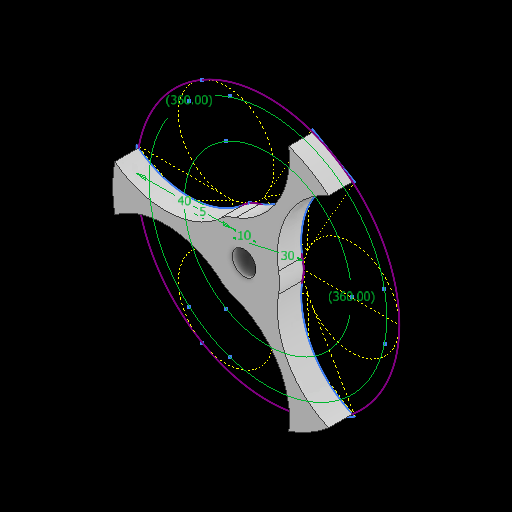
# Autodesk Inventor part: Combine mk1
Saved by Autodesk Inventor 2025 (Build 290162000, 162)
## iProperties
Created: 2024-09-10
Part Number: Combine mk1
Material: Generic
Document SubType Name: Modeling
Designer: Trevor
Density: 1 g/cm^3
Appearance: Default
Author: Trevor
Autodesk Inventor part; units mm, degrees
ref_plane "YZ Plane" through (0, 0, 0) normal (1, 0, 0) x (0, 1, 0)
ref_plane "XZ Plane" through (0, 0, 0) normal (0, 1, 0) x (-1, 0, 0)
ref_plane "XY Plane" through (0, 0, 0) normal (0, 0, 1) x (1, 0, 0)
sketch "Sketch1" plane through (0, 0, 0) normal (0, 0, 1) x (1, 0, 0)
  circle A0 centre (0, 0) radius 15
  circle A1 centre (0, 0) radius 55
  line L0 (15, 0) -> (55, 0) construction
  circle A2 centre (35, 0) radius 20 construction
  circle A3 centre (-17.5, 30.310889) radius 20 construction
  circle A4 centre (-17.5, -30.310889) radius 20 construction
  line L1 (0, 0) -> (-10.833994, 10.374226)
  line L2 (0, 0) -> (27.5, -47.631397)
  line L3 (0, 0) -> (-55, 0) construction
  line L4 (0, 0) -> (27.5, 47.631397)
  line L5 (17.5, 30.310889) -> (27.5, 47.631397) construction
  line L6 (-1.432373, 18.147489) -> (18.567627, 52.788505) construction
  line L7 (18.567627, 52.788505) -> (36.432373, 42.47429) construction
  line L8 (36.432373, 42.47429) -> (16.432373, 7.833273) construction
  line L9 (16.432373, 7.833273) -> (-1.432373, 18.147489) construction
  line L10 (-1.432373, 18.147489) -> (36.432373, 42.47429) construction
  line L11 (18.567627, 52.788505) -> (16.432373, 7.833273) construction
  line L12 (-1.48905, -18.180212) -> (18.51095, -52.821228) construction
  line L13 (18.51095, -52.821228) -> (36.48905, -42.441567) construction
  line L14 (36.48905, -42.441567) -> (16.48905, -7.80055) construction
  line L15 (16.48905, -7.80055) -> (-1.48905, -18.180212) construction
  line L16 (-1.48905, -18.180212) -> (36.48905, -42.441567) construction
  line L17 (18.51095, -52.821228) -> (16.48905, -7.80055) construction
  line L18 (-55.008072, 10.310889) -> (-15, 10.310889) construction
  line L19 (-15, 10.310889) -> (-15, -10.310889) construction
  line L20 (-15, -10.310889) -> (-55.008072, -10.310889) construction
  line L21 (-55.008072, -10.310889) -> (-55.008072, 10.310889)
  line L22 (-55.008072, 10.310889) -> (-15, -10.310889) construction
  line L23 (-15, 10.310889) -> (-55.008072, -10.310889) construction
  line L24 (-39.117828, -2.5) -> (-30.890244, -2.5) construction
  line L25 (-30.890244, -2.5) -> (-30.890244, 2.5) construction
  line L26 (-30.890244, 2.5) -> (-39.117828, 2.5) construction
  line L27 (-39.117828, 2.5) -> (-39.117828, -2.5) construction
  line L28 (-39.117828, -2.5) -> (-30.890244, 2.5) construction
  line L29 (-30.890244, -2.5) -> (-39.117828, 2.5) construction
  arc A5 (-10.89429, -10.310889) -> (-55.008072, -10.310889) centre (-32.951181, -37.548278) ccw
  line L30 (-55.008072, 10.310889) -> (-55.008072, -10.310889) construction
  arc A6 (-55.008072, 10.310889) -> (-10.833994, 10.374226) centre (-32.959623, 37.256893) ccw
  line L31 (-55.008072, 10.310889) -> (-55.008072, -10.310889) construction
  arc A7 (18.574544, -52.793832) -> (-3.567347, -14.569627) centre (-15.785604, -47.172317) ccw
  line L32 (36.433528, -42.482943) -> (18.574544, -52.793832)
  arc A8 (14.376637, -4.279288) -> (36.433528, -42.482943) centre (48.993353, -9.762421) ccw
  circle A9 centre (0, 0) radius 15
  arc A10 (36.433528, 42.482943) -> (14.401341, 4.195401) centre (48.745227, 9.915425) ccw
  line L33 (18.574544, 52.793832) -> (36.433528, 42.482943)
  arc A11 (-3.482347, 14.590177) -> (18.574544, 52.793832) centre (-16.042172, 47.310699) ccw
  circle A12 centre (0, 0) radius 15
  circle A13 centre (0, 0) radius 5
  point P0 (-27.5, 47.631397)
  point P1 (-27.5, -47.631397)
  point P2 (17.5, -30.310889)
  point P3 (-35.004036, 0)
  point P4 (-7.5, 12.990381)
  point P5 (-7.5, -12.990381)
  point P6 (-54.150171, 9.631146)
  point P7 (-54.1491, -9.637168)
  point P8 (-3.567347, -14.569627)
  point P9 (18.734269, -51.710997)
  point P10 (35.420582, -42.075912)
  point P11 (14.376637, -4.279288)
  point P12 (14.401341, 4.195401)
  point P13 (35.415903, 42.079851)
  point P14 (18.728517, 51.71308)
  point P15 (-3.482347, 14.590177)
  dimension "d0" = 30
  dimension "d1" = 40
  dimension "d4" = 360
  dimension "d6" = 5
  dimension "d9" = 360
  dimension "d11" = 10
  constraints: 68 end point, 25 point on circle, 11 centre point, 9 midpoint, 9 parallel, 4 perpendicular, 4 point on line, 3 coincident, 2 horizontal, 1 horizontal alignment, 1 tangent, 56 other
  measures "d0" diameter of A0
  measures "d1" radial gap between concentric circles of A0 A1
  measures "d6" distance of L25.end L24.end
  measures "d11" radial gap between concentric circles of A0 A13
sketch "Sketch1 outline for Extrusion1" plane through (0, 0, 0) normal (0, 0, 1) x (1, 0, 0)
  arc A0 (-10.833994, 10.374226) -> (-54.150171, 9.631146) centre (-32.959623, 37.256893) cw
  arc A1 (-3.482347, 14.590177) -> (-10.833994, 10.374226) centre (0, 0) ccw
  arc A2 (-54.150171, 9.631146) -> (-54.1491, -9.637168) centre (0, 0) ccw
  arc A3 (18.728517, 51.71308) -> (-3.482347, 14.590177) centre (-16.042172, 47.310699) cw
  arc A4 (-54.1491, -9.637168) -> (-10.89429, -10.310889) centre (-32.951181, -37.548278) cw
  arc A5 (35.415903, 42.079851) -> (18.728517, 51.71308) centre (0, 0) ccw
  arc A6 (-10.89429, -10.310889) -> (-3.567347, -14.569627) centre (0, 0) ccw
  arc A7 (14.401341, 4.195401) -> (35.415903, 42.079851) centre (48.745227, 9.915425) cw
  arc A8 (-3.567347, -14.569627) -> (18.734269, -51.710997) centre (-15.785604, -47.172317) cw
  arc A9 (14.376637, -4.279288) -> (14.401341, 4.195401) centre (0, 0) ccw
  arc A10 (18.734269, -51.710997) -> (35.420582, -42.075912) centre (0, 0) ccw
  arc A11 (35.420582, -42.075912) -> (14.376637, -4.279288) centre (48.993353, -9.762421) cw
  circle A12 centre (0, 0) radius 5
extrude "Extrusion1" add sketch "Sketch1 outline for Extrusion1" along normal blind 10
body "Solid1"
